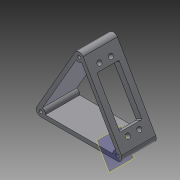
# Autodesk Inventor part: ServoHousing
Saved by Autodesk Inventor 2014 SP1 (Build 180222100, 222)
## iProperties
Created: 2014-11-03
Part Number: ServoHousing
Material: Generic
Document SubType Name: Modeling
Designer: rawrdong
Density: 1 g/cm^3
Appearance: Default
Author: rawrdong
Autodesk Inventor part; units mm, degrees
ref_plane "YZ Plane" through (0, 0, 0) normal (1, 0, 0) x (0, 1, 0)
ref_plane "XZ Plane" through (0, 0, 0) normal (0, 1, 0) x (-1, 0, 0)
ref_plane "XY Plane" through (0, 0, 0) normal (0, 0, 1) x (1, 0, 0)
sketch "Sketch2" plane through (0, 0, 0) normal (0, 1, 0) x (-1, 0, 0)
  circle A0 centre (0, 38.6825) radius 1.425
  circle A1 centre (0, 38.6825) radius 4
  circle A2 centre (-33.5, -19.3412) radius 1.425
  circle A3 centre (-33.5, -19.3412) radius 4
  circle A4 centre (33.5, -19.3412) radius 1.425
  circle A5 centre (33.5, -19.3412) radius 4
  line L0 (-36.9641, -17.3412) -> (-3.4641, 40.6825)
  line L1 (-2.4173, 35.4955) -> (-31.9487, -15.6543)
  line L2 (-33.5, -23.3412) -> (33.5, -23.3412)
  line L3 (36.9641, -17.3412) -> (3.4641, 40.6825)
  line L4 (-29.5314, -19.8412) -> (29.5314, -19.8412)
  line L5 (31.9487, -15.6543) -> (2.4173, 35.4955)
  line L6 (0, -23.3412) -> (0, -19.8412) construction
  line L7 (20.2141, 11.6706) -> (17.183, 9.9206) construction
  line L8 (-17.183, 9.9206) -> (-20.2141, 11.6706) construction
  point P0 (0, 0)
  point P1 (0, 0)
  dimension "d21" = 360
  dimension "d23" = 67
  dimension "d24" = 2.85
  dimension "d25" = 8
  dimension "d30" = 3.5
  constraints: 18 end point, 12 point on circle, 6 centre point, 6 midpoint, 6 tangent, 4 coincident, 3 parallel, 2 equal length, 1 horizontal, 1 vertical alignment, 13 other
  measures "d23" distance of A4.centre A2.centre
  measures "d24" diameter of A2
  measures "d25" diameter of A3
  measures "d30" distance between parallel lines of L0 L1
extrude "Extrusion3" add sketch "Sketch2" along normal blind 30 contours A1 | A1 L3 A5 L5 | A1 L1 A3 L0 | A5 | A3 | A5 L2 A3 L4
sketch "Servo1" plane through (36.9641, 0, -17.3412) normal (0.8660254, 0, 0.5) x (0.5, 0, -0.8660254)
  line L0 (-67, 30) -> (0, 30) projected
  line L1 (-53.6125, 24.65) -> (-13.3875, 24.65)
  line L2 (-13.3875, 24.65) -> (-13.3875, 5.35)
  line L3 (-13.3875, 5.35) -> (-53.6125, 5.35)
  line L4 (-53.6125, 5.35) -> (-53.6125, 24.65)
  circle A0 centre (-8.6975, 20.025) radius 2.025
  circle A1 centre (-8.6975, 9.975) radius 2.025
  line L5 (-33.5, 30) -> (-33.5, -15.5284)
  line L6 (-13.3875, 15) -> (-53.6125, 15) construction
  circle A2 centre (-58.3025, 20.025) radius 2.025
  circle A3 centre (-58.3025, 9.975) radius 2.025
  line L7 (0, 0) -> (0, 30) projected
  point P0 (-33.5, 0)
  point P1 (-33.5, 5.35)
  point P2 (0, 15)
  dimension "d43" = 4.05
  dimension "d44" = 19.3
  dimension "d45" = 40.225
  dimension "d46" = 6
  dimension "d47" = 49.605
  constraints: 12 end point, 5 midpoint, 4 centre point, 3 parallel, 3 symmetric about line, 1 equal radius, 1 horizontal, 1 horizontal alignment, 1 perpendicular, 1 point on line, 2 other
  measures "d43" diameter of A0
  measures "d44" distance of L3.end L1.start
  measures "d45" distance of L2.end L3.end
  measures "d47" diameter of A0.centre L5
extrude "Extrusion4" cut sketch "Servo1" against normal blind 27 contours L1 L5 L3 L4 | L1 L2 L3 L5
extrude "Extrusion5" cut sketch "Servo1" against normal up to next contours A0 | A1 | A2 | A3
fillet "Fillet4" radius 0.8 4 edges at (8.6423, 24.65, 28.2136) (8.6423, 5.35, 28.2136) (28.7548, 5.35, -6.6223) (28.7548, 24.65, -6.6223)
ref_plane "Work Plane1" through (31.683, 0, -15.1941) normal (-0.8660254, 0, -0.5) x (-0.5, 0, 0.8660254)
sketch "Sketch7" plane through (31.683, 0, -15.1941) normal (-0.8660254, 0, -0.5) x (-0.5, 0, 0.8660254)
  line L0 (49.1125, 6.15) -> (49.1125, 23.85) projected
  line L1 (48.3125, 24.65) -> (9.6875, 24.65) projected
  arc A0 (49.1125, 23.85) -> (48.3125, 24.65) centre (48.3125, 23.85) ccw projected
  arc A1 (48.3125, 5.35) -> (49.1125, 6.15) centre (48.3125, 6.15) ccw projected
  line L2 (9.6875, 5.35) -> (48.3125, 5.35) projected
  arc A2 (8.8875, 6.15) -> (9.6875, 5.35) centre (9.6875, 6.15) ccw projected
  line L3 (8.8875, 23.85) -> (8.8875, 6.15) projected
  arc A3 (9.6875, 24.65) -> (8.8875, 23.85) centre (9.6875, 23.85) ccw projected
  line L4 (9.6875, 27.15) -> (48.3125, 27.15)
  arc A4 (51.6125, 23.85) -> (48.3125, 27.15) centre (48.3125, 23.85) ccw
  line L5 (51.6125, 23.85) -> (51.6125, 6.15)
  arc A5 (48.3125, 2.85) -> (51.6125, 6.15) centre (48.3125, 6.15) ccw
  line L6 (48.3125, 2.85) -> (9.6875, 2.85)
  arc A6 (6.3875, 6.15) -> (9.6875, 2.85) centre (9.6875, 6.15) ccw
  line L7 (6.3875, 6.15) -> (6.3875, 23.85)
  arc A7 (9.6875, 27.15) -> (6.3875, 23.85) centre (9.6875, 23.85) ccw
  line L8 (6.3875, 23.85) -> (-2.5584, 23.85)
  line L9 (-2.5584, 23.85) -> (-2.5584, 6.15)
  line L10 (6.3875, 6.15) -> (-2.5584, 6.15)
  line L11 (29, 5.35) -> (29, 24.65) construction
  line L12 (51.6125, 23.85) -> (60.5584, 23.85)
  line L13 (60.5584, 23.85) -> (60.5584, 6.15)
  line L14 (51.6125, 6.15) -> (60.5584, 6.15)
  circle A8 centre (4.1975, 20.025) radius 2.025 projected
  circle A9 centre (4.1975, 9.975) radius 2.025 projected
  circle A10 centre (53.8025, 9.975) radius 2.025 projected
  circle A11 centre (53.8025, 20.025) radius 2.025 projected
  dimension "d82" = 2.5
  constraints: 22 end point, 8 point on circle, 4 centre point, 3 perpendicular, 2 horizontal, 2 midpoint, 1 vertical, 8 other
  measures "d82" distance between parallel lines of L4 L1
extrude "Extrusion8" add sketch "Sketch7" along normal blind 2
fillet "Fillet6" radius 2 4 edges at (27.6232, 23.85, -10.1624) (5.0107, 23.85, 29.0036) (5.0107, 6.15, 29.0036) (27.6232, 6.15, -10.1624)
chamfer "Chamfer2" distance 2 angle 45 14 edges at (17.183, 27.15, 9.9206) (6.6061, 26.5886, 28.2403) (5.6306, 24.1903, 29.9299) (3.745, 23.85, 33.1959) (27.7599, 26.5886, -8.3991) (28.7354, 24.1903, -10.0887) (30.621, 23.85, -13.3547) (17.183, 2.85, 9.9206) (27.7599, 3.4114, -8.3991) (28.7354, 5.8097, -10.0887) (30.621, 6.15, -13.3547) (6.6061, 3.4114, 28.2403) (5.6306, 5.8097, 29.9299) (3.745, 6.15, 33.1959)
body "Solid2"
body "Solid3"
